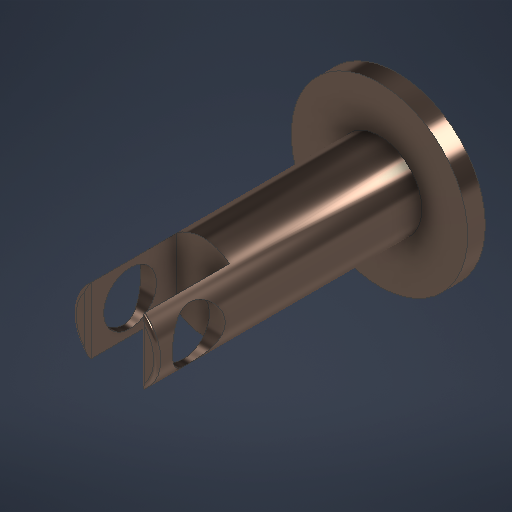
# Autodesk Inventor part: Part1final
Saved by Autodesk Inventor 2026 (Build 300175050, 175E)
## iProperties
Created: 2026-05-04
Part Number: Part1final
Material: Steel, Carbon
Document SubType Name: Modeling
Designer: ptp527
Mass: 266782 g
Surface Area: 10034.4 cm^2
Volume: 33984.9 cm^3
Density: 7.85 g/cm^3
Appearance: Semi-Polished
Author: ptp527
Autodesk Inventor part; units mm, degrees
ref_plane "YZ Plane" through (0, 0, 0) normal (1, 0, 0) x (0, 1, 0)
ref_plane "XZ Plane" through (0, 0, 0) normal (0, 1, 0) x (-1, 0, 0)
ref_plane "XY Plane" through (0, 0, 0) normal (0, 0, 1) x (1, 0, 0)
sketch "Sketch1" plane through (0, 0, 0) normal (0, 0, 1) x (1, 0, 0)
  circle A0 centre (0, 0) radius 250
  dimension "d0" = 500
  constraints: 1 centre point, 1 coincident
  measures "d0" diameter of A0
extrude "Extrusion1" add sketch "Sketch1" along normal blind 50
sketch "Sketch2" plane through (0, 0, 50) normal (0, 0, 1) x (1, 0, 0)
  circle A0 centre (0, 0) radius 120
  dimension "d3" = 240
  constraints: 1 centre point, 1 coincident
  measures "d3" diameter of A0
extrude "Extrusion2" add sketch "Sketch2" along normal blind 750
sketch "Sketch3" plane through (0, 0, 800) normal (0, 0, 1) x (1, 0, 0)
  line L0 (-75, -121) -> (75, -121)
  line L1 (75, -121) -> (75, 121)
  line L2 (75, 121) -> (-75, 121)
  line L3 (-75, 121) -> (-75, -121)
  line L4 (-75, -121) -> (75, 121) construction
  line L5 (75, -121) -> (-75, 121) construction
  point P0 (0, 0)
  dimension "d6" = 150
  dimension "d7" = 150
  dimension "d8" = 121
  constraints: 12 end point, 2 midpoint, 2 parallel, 1 horizontal, 1 perpendicular
  measures "d6" distance of L1.end L2.end
  measures "d7" distance between parallel lines of L1 L3
  measures "d8" distance from line of L0 point (0, 0)
extrude "Extrusion3" cut sketch "Sketch3" against normal blind 250
sketch "Sketch4" plane through (-75, -93.675, 800) normal (1, 0, 0) x (0, 0, -1)
  circle A0 centre (118.0956, 93.675) radius 75
  point P0 (800, 93.675)
  dimension "d11" = 150
  constraints: 1 centre point
  measures "d11" diameter of A0
extrude "Extrusion4" cut sketch "Sketch4" along normal mid plane 500
fillet "Fillet1" radius 10 5 edges at (-120, 0, 800) (-75, 0, 800) (75, 0, 800) (108.1665, -51.9615, 800) (108.1665, 51.9615, 800)
body "Solid1"
